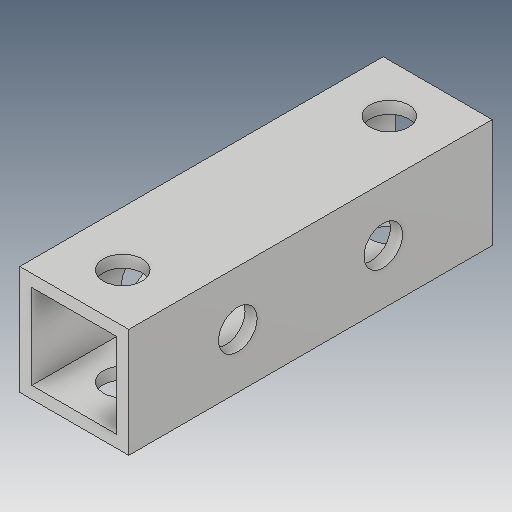
# Autodesk Inventor part: 肩ピッチ固定角柱B_9×9
Saved by Autodesk Inventor 2019.4 (Build 234330000, 330)
## iProperties
Created: 2019-06-28
Part Number: 肩ピッチ固定角柱B_9×9
Material: アルミニウム 2014-T6
Document SubType Name: Modeling
Designer: 長谷川翔一
Mass: 2.6777 g
Surface Area: 19.84 cm^2
Volume: 0.96 cm^3
Density: 2.78927 g/cm^3
Appearance: サテン
Author: 長谷川翔一
Autodesk Inventor part; units mm, degrees
ref_plane "YZ Plane" through (0, 0, 0) normal (1, 0, 0) x (0, 1, 0)
ref_plane "XZ Plane" through (0, 0, 0) normal (0, 1, 0) x (-1, 0, 0)
ref_plane "XY Plane" through (0, 0, 0) normal (0, 0, 1) x (1, 0, 0)
sketch "スケッチ1" plane through (0, 0, 0) normal (0, 0, 1) x (1, 0, 0)
  line L0 (4.5, -4.5) -> (-4.5, -4.5)
  line L1 (-4.5, -4.5) -> (-4.5, 4.5)
  line L2 (-4.5, 4.5) -> (4.5, 4.5)
  line L3 (4.5, 4.5) -> (4.5, -4.5)
  line L4 (4.5, -4.5) -> (-4.5, 4.5) construction
  line L5 (-4.5, -4.5) -> (4.5, 4.5) construction
  line L6 (3.5, 3.5) -> (-3.5, 3.5)
  line L7 (-3.5, 3.5) -> (-3.5, -3.5)
  line L8 (-3.5, -3.5) -> (3.5, -3.5)
  line L9 (3.5, -3.5) -> (3.5, 3.5)
  point P0 (0, 0)
  dimension "d0" = 9
  dimension "d1" = 9
  dimension "d2" = 1
  constraints: 20 end point, 4 parallel, 2 midpoint, 2 perpendicular, 1 horizontal, 3 other
  measures "d0" distance of L1.end L2.end
  measures "d1" distance of L0.end L1.end
  measures "d2" distance between parallel lines of L2 L6
extrude "押し出し1" add sketch "スケッチ1" along normal blind 30
sketch "スケッチ2" plane through (-4.5, 4.5, 0) normal (0, 1, 0) x (1, 0, 0)
  line L0 (0, 0) -> (9, 0) projected
  line L1 (0, 0) -> (0, -30) projected
  line L2 (9, -30) -> (0, -30) projected
  line L3 (9, 0) -> (9, -30) projected
  line L4 (4.5, -30) -> (4.5, 0) construction
  line L5 (4.5, -15) -> (0, -15) construction
  circle A0 centre (4.5, -26) radius 1.6
  circle A1 centre (4.5, -4) radius 1.6
  dimension "d5" = 3.2
  dimension "d6" = 4
  constraints: 4 end point, 3 midpoint, 2 centre point, 1 point on line, 1 symmetric about line, 1 vertical, 1 other
  measures "d5" diameter of A0
  measures "d6" distance from line of A0.centre L2
extrude "押し出し2" cut sketch "スケッチ2" against normal through all contours A0 | A1
sketch "スケッチ3" plane through (4.5, -4.5, 0) normal (1, 0, 0) x (0, 0, -1)
  line L0 (0, 9) -> (0, 0) projected
  line L1 (0, 9) -> (-30, 9) projected
  line L2 (-30, 0) -> (-30, 9) projected
  line L3 (0, 0) -> (-30, 0) projected
  line L4 (-30, 4.5) -> (0, 4.5) construction
  line L5 (-15, 4.5) -> (-15, 9) construction
  circle A0 centre (-21, 4.5) radius 1.6
  circle A1 centre (-9, 4.5) radius 1.6
  line L6 (-9, 4.5) -> (-21, 4.5)
  line L7 (0, 9) -> (-30, 9) projected
  dimension "d9" = 3.2
  dimension "d13" = 12
  constraints: 6 end point, 5 midpoint, 2 centre point, 2 horizontal, 1 point on line, 1 symmetric about line, 1 vertical alignment, 1 other
  measures "d9" diameter of A0
  measures "d13" distance of L6.start L6.end
extrude "押し出し3" cut sketch "スケッチ3" against normal through all contours A0 | A1
